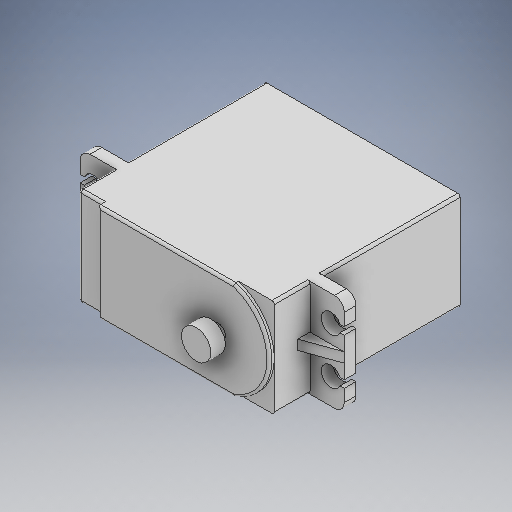
# Autodesk Inventor part: Servo996R_180º
Saved by Autodesk Inventor 2025.2 (Build 292293000, 293)
## iProperties
Created: 2025-04-06
Part Number: Servo996R_180º
Material: Generic
Document SubType Name: Modeling
Designer: Tiago
Density: 1 g/cm^3
Appearance: Default
Author: Tiago
Autodesk Inventor part; units mm, degrees
ref_plane "YZ Plane" through (0, 0, 0) normal (1, 0, 0) x (0, 1, 0)
ref_plane "XZ Plane" through (0, 0, 0) normal (0, 1, 0) x (-1, 0, 0)
sketch "Sketch1" plane through (0, 0, 0) normal (0, 0, 1) x (1, 0, 0)
  line L0 (-20, -10) -> (20, -10)
  line L1 (20, -10) -> (20, 10)
  line L2 (20, 10) -> (-20, 10)
  line L3 (-20, 10) -> (-20, -10)
  line L4 (-20, -10) -> (20, 10) construction
  line L5 (20, -10) -> (-20, 10) construction
  point P0 (0, 0)
  dimension "d0" = 40
  dimension "d1" = 20
  constraints: 12 end point, 2 midpoint, 2 parallel, 1 horizontal, 1 perpendicular
  measures "d0" distance of L2.end L1.end
  measures "d1" distance of L0.end L1.end
extrude "Extrusion1" add sketch "Sketch1" along normal blind 39
ref_plane "Work Plane1" through (0, 0, 28.3) normal (0, 0, 1) x (1, 0, 0)
sketch "Sketch2" plane through (0, 0, 28.3) normal (0, 0, 1) x (1, 0, 0)
  line L0 (20, -10) -> (-20, -10) projected
  line L1 (-20, -10) -> (-20, 10) projected
  line L2 (-20, 10) -> (20, 10) projected
  line L3 (20, 10) -> (20, -10) projected
  line L4 (-27, -10) -> (27, -10)
  line L5 (27, -10) -> (27, 10)
  line L6 (27, 10) -> (-27, 10)
  line L7 (-27, 10) -> (-27, -10)
  line L8 (-27, -10) -> (27, 10) construction
  line L9 (27, -10) -> (-27, 10) construction
  line L10 (-27, -4.7082) -> (-24.3, -4.7082) construction
  line L11 (-24.3, -4.7) -> (-24.3, 4.7) construction
  arc A0 (-26.154, 3.95) -> (-26.154, 5.45) centre (-24.3, 4.7) ccw
  arc A1 (-26.1507, -5.4582) -> (-26.1573, -3.9582) centre (-24.3, -4.7) ccw
  line L12 (0, 13.3238) -> (0, -12.3222) construction
  arc A2 (26.154, 5.45) -> (26.154, 3.95) centre (24.3, 4.7) ccw
  arc A3 (26.1573, -3.9582) -> (26.1507, -5.4582) centre (24.3, -4.7) ccw
  line L13 (-27, 3.95) -> (-27, 5.45)
  line L14 (-27, -5.4582) -> (-27, -3.9582)
  line L15 (-27, 5.45) -> (-26.154, 5.45)
  line L16 (-27, 3.95) -> (-26.154, 3.95)
  line L17 (-27, -3.9582) -> (-26.1573, -3.9582)
  line L18 (-27, -5.4582) -> (-26.1507, -5.4582)
  line L19 (27, 5.45) -> (26.154, 5.45)
  line L20 (27, 3.95) -> (26.154, 3.95)
  line L21 (27, -3.9582) -> (26.1573, -3.9582)
  line L22 (27, -5.4582) -> (26.1507, -5.4582)
  point P0 (0, 0)
  point P1 (24.3, -4.7082)
  point P2 (-27, 4.7)
  dimension "d5" = 54
  dimension "d13" = 2.7
  dimension "d14" = 9.4
  dimension "furos" = 4
  dimension "d16" = 4
  dimension "d29" = 1.5
  dimension "d30" = 1.5
  constraints: 38 end point, 12 symmetric about line, 8 point on circle, 5 parallel, 4 centre point, 4 midpoint, 4 point on line, 3 coincident, 3 horizontal, 2 perpendicular, 1 vertical, 2 other
  measures "d5" distance of L6.end L5.end
  measures "d13" distance of L10.start L10.end
  measures "d14" distance of L11.start L11.end
  measures "furos" diameter of A0
  measures "d16" diameter of A1
  measures "d29" distance of L13.start L13.end
  measures "d30" distance of L14.start L14.end
extrude "Extrusion2" add sketch "Sketch2" along normal blind 2.4 contours L3 L6 L5 L19 A2 L20 L21 A3 L22 L4 | L4 L7 L18 A1 L17 L16 A0 L15 L6 L1 | L22 A3 L21 L5 | L7 L17 A1 L18 | L5 L20 A2 L19 | L15 A0 L16 L7
sketch "Sketch3" plane through (0, 0, 0) normal (0, 1, 0) x (-1, 0, 0)
  line L0 (-27, 28.3) -> (-27, 30.7) projected
  line L1 (-27, 30.7) -> (-20, 30.7) projected
  line L2 (-20, 30.7) -> (-20, 39) projected
  line L3 (-20, 39) -> (20, 39) projected
  line L4 (20, 39) -> (20, 30.7) projected
  line L5 (20, 30.7) -> (27, 30.7) projected
  line L6 (27, 30.7) -> (27, 28.3) projected
  line L7 (27, 28.3) -> (20, 28.3) projected
  line L8 (20, 28.3) -> (20, 0) projected
  line L9 (20, 0) -> (-20, 0) projected
  line L10 (-20, 0) -> (-20, 28.3) projected
  line L11 (-20, 28.3) -> (-27, 28.3) projected
  line L12 (20, 30.7) -> (20, 33.2)
  line L13 (20, 33.2) -> (27, 30.7)
  line L14 (27, 30.7) -> (20, 30.7)
  line L15 (0, 28.3) -> (0, 40.3429)
  line L16 (-20, 39) -> (-20, 30.7)
  line L17 (-20, 30.7) -> (-27, 30.7)
  line L18 (-20, 30.7) -> (-20, 33.2)
  line L19 (-20, 33.2) -> (-27, 30.7)
  line L20 (-27, 30.7) -> (-20, 30.7)
  point P0 (0, 0)
  dimension "d8" = 2.5
  constraints: 18 end point, 2 point on line, 1 collinear, 1 symmetric about line, 1 vertical
  measures "d8" distance of L4.end L12.end
extrude "Extrusion4" add sketch "Sketch3" along normal mid plane 2 contours L19 L2 L1 | L13 L5 L4
extrude "Extrusion5" cut sketch "Sketch2" along normal up to surface (2.4 mm away) contours L22 A3 L21 L5 | L7 L17 A1 L18 | L5 L20 A2 L19 | L15 A0 L16 L7
sketch "Sketch4" plane through (0, 0, 39) normal (0, 0, 1) x (1, 0, 0)
  line L0 (20, 10) -> (20, -10) construction
  line L1 (20, 0) -> (9.5, 0) construction
  circle A0 centre (9.5, 0) radius 1.5
  point P0 (0, 0)
  dimension "d19" = 10.5
  dimension "d20" = 3
  constraints: 2 end point, 1 centre point, 1 coincident, 1 horizontal, 1 midpoint
  measures "d19" distance of L1.start L1.end
  measures "d20" diameter of A0
extrude "Extrusion6" add sketch "Sketch4" along normal blind 1.5
sketch "Sketch5" plane through (9.5, 0, 40.5) normal (0, 0, 1) x (1, 0, 0)
  circle A0 centre (0, 0) radius 3
  point P0 (-9.5, 0)
  dimension "d23" = 6
  constraints: 1 centre point
  measures "d23" diameter of A0
extrude "Extrusion7" add sketch "Sketch5" along normal blind 3
sketch "Sketch6" plane through (0, 0, 39) normal (0, 0, 1) x (1, 0, 0)
  circle A0 centre (9.5, 0) radius 1.5 projected
  line L0 (20, 10) -> (20, -10) projected
  line L1 (20, -10) -> (-20, -10) projected
  line L2 (-20, -10) -> (-20, 10) projected
  line L3 (-20, 10) -> (20, 10) projected
  line L4 (-20, 10) -> (-15, 10)
  line L5 (-15, 10) -> (-15, -10)
  line L6 (-15, -10) -> (-20, -10)
  line L7 (-20, -10) -> (-20, 10)
  arc A1 (12.7016, -10) -> (12.7016, 10) centre (9.5, 0) ccw
  point P0 (0, 0)
  point P1 (20, 0)
  dimension "d26" = 5
  constraints: 8 end point, 4 point on line, 2 perpendicular, 2 point on circle, 1 centre point, 1 coincident, 1 collinear, 1 tangent
  measures "d26" distance of L2.end L4.end
extrude "Extrusion8" cut sketch "Sketch6" against normal blind 1 contours L0 A1 L3 | L0 L1 A1 | L5 L1 L2 L3
fillet "Fillet1" radius 2 4 edges at (-27, -10, 29.5) (-27, 10, 29.5) (27, -10, 29.5) (27, 10, 29.5)
fillet "Fillet2" radius 0.5 15 edges at (-1.1492, -10, 39) (20, 0, 39) (-1.1492, 10, 39) (-15, 0, 39) (-17.5, -10, 38) (-20, 0, 38) (-17.5, 10, 38) (20, 10, 34.35) (20, -10, 34.35) (20, -10, 14.15) (20, 10, 14.15) (-20, -10, 14.15) (-20, -10, 34.35) (-20, 10, 34.35) (-20, 10, 14.15)
equation "\"d16\" = furos"
body "Solid1"
